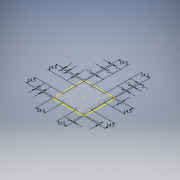
# Autodesk Inventor part: Cover
Saved by Autodesk Inventor 2016 (Build 200138000, 138)
## iProperties
Created: 2016-04-15
Part Number: Cover
Material: Generic
Document SubType Name: Modeling
Designer: Andres
Density: 1 g/cm^3
Appearance: Clear - Light
Author: Andres
Autodesk Inventor part; units mm, degrees
ref_plane "YZ Plane" through (0, 0, 0) normal (1, 0, 0) x (0, 1, 0)
ref_plane "XZ Plane" through (0, 0, 0) normal (0, 1, 0) x (-1, 0, 0)
ref_plane "XY Plane" through (0, 0, 0) normal (0, 0, 1) x (1, 0, 0)
sketch "Sketch1" plane through (0, 0, 0) normal (0, 0, 1) x (1, 0, 0)
  line L0 (-25, 25) -> (25, 25)
  line L1 (25, 25) -> (25, -25)
  line L2 (25, -25) -> (-25, -25)
  line L3 (-25, -25) -> (-25, 25)
  point P0 (0, 0)
  point P1 (-25, 0)
  point P2 (0, 25)
  dimension "d0" = 50
  dimension "d1" = 50
  constraints: 8 end point, 2 midpoint, 2 parallel, 1 horizontal, 1 horizontal alignment, 1 perpendicular, 1 vertical alignment
  measures "d0" distance of L0.end L1.end
  measures "d1" distance of L0.start L0.end
extrude "Extrusion1" add sketch "Sketch1" along normal blind 4
chamfer "Chamfer1" distance 4 distance2 2 1 edges at (0, -25, 4) measured on face at (0, -24.5, 4)
chamfer "Chamfer2" distance 4 distance2 2 1 edges at (25, 2, 4) measured on face at (24.5, 2, 4)
chamfer "Chamfer3" distance 4 distance2 2 1 edges at (-25, 2, 4) measured on face at (-24.5, 2, 4)
chamfer "Chamfer4" distance 4 distance2 2 1 edges at (0, 25, 4) measured on face at (0, 24.5, 4)
sketch "Sketch2" plane through (0, 0, 0) normal (0, 0, -1) x (-1, 0, 0)
  point P0 (0, 0)
sketch "Sketch3" plane through (0, 0, 0) normal (0, 0, -1) x (-1, 0, 0)
  point P0 (0, 0)
sketch "Sketch4" plane through (0, 0, 0) normal (0, 0, -1) x (-1, 0, 0)
  point P0 (0, 0)
sketch "Sketch5" plane through (0, 0, 0) normal (0, 0, -1) x (-1, 0, 0)
  line L0 (25, -25) -> (25, 25) projected
  line L1 (25, 25) -> (-25, 25) projected
  line L2 (-25, 25) -> (-25, -25) projected
  line L3 (-25, -25) -> (25, -25) projected
  line L4 (25, -25) -> (21, -21) projected
  point P0 (0, 0)
  point P1 (23, 23)
  point P2 (-23, 23)
  point P3 (-23, -23)
  point P4 (-23, -10.5)
  point P5 (-23, 10.5)
  point P6 (10.5, 23)
  point P7 (-10.5, 23)
  point P8 (23, 10.5)
  point P9 (23, -10.5)
  point P10 (10.5, -23)
  point P11 (-10.5, -23)
  point P12 (23, -23)
  dimension "d18" = 2
  dimension "d19" = 2
  dimension "d20" = 2
  dimension "d21" = 2
  dimension "d22" = 2
  dimension "d23" = 2
  dimension "d24" = 2
  dimension "d25" = 2
  dimension "d26" = 2
  dimension "d27" = 2
  dimension "d28" = 2
  dimension "d29" = 2
  dimension "d30" = 2
  dimension "d31" = 2
  dimension "d32" = 14.5
  dimension "d33" = 14.5
  dimension "d34" = 14.5
  dimension "d35" = 14.5
  dimension "d36" = 14.5
  dimension "d37" = 14.5
  dimension "d38" = 14.5
  dimension "d39" = 14.5
  constraints: 1 midpoint
  measures "d18" distance from line of L0 point (23, 23)
  measures "d19" distance from line of L1 point (23, 23)
  measures "d20" distance from line of L2 point (-23, 23)
  measures "d21" distance from line of L1 point (10.5, 23)
  measures "d22" distance from line of L1 point (-10.5, 23)
  measures "d23" distance from line of L1 point (-23, 23)
  measures "d24" distance from line of L0 point (23, 10.5)
  measures "d25" distance from line of L0 point (23, -10.5)
  measures "d26" distance from line of L3 point (10.5, -23)
  measures "d27" distance from line of L3 point (-10.5, -23)
  measures "d28" distance from line of L2 point (-23, 10.5)
  measures "d29" distance from line of L2 point (-23, -10.5)
  measures "d30" distance from line of L3 point (-23, -23)
  measures "d31" distance from line of L2 point (-23, -23)
  measures "d32" distance from line of L1 point (-23, 10.5)
  measures "d33" distance from line of L3 point (-23, -10.5)
  measures "d34" distance from line of L2 point (-10.5, 23)
  measures "d35" distance from line of L0 point (10.5, 23)
  measures "d36" distance from line of point (23, 10.5) L1
  measures "d37" distance from line of L3 point (23, -10.5)
  measures "d38" distance from line of L0 point (10.5, -23)
  measures "d39" distance from line of L2 point (-10.5, -23)
sketch "Sketch6" plane through (0, 0, 0) normal (0, 0, -1) x (-1, 0, 0)
  point P0 (23, 23)
  point P1 (-23, 23)
  point P2 (-23, -23)
  point P3 (-23, -10.5)
  point P4 (-23, 10.5)
  point P5 (10.5, 23)
  point P6 (-10.5, 23)
  point P7 (23, 10.5)
  point P8 (10.5, -23)
  point P9 (-10.5, -23)
  point P10 (23, -23)
  point P11 (23, -10.5)
hole "Hole1" at (-23, 23, 0) at (23, 23, 0) at (23, -23, 0) at (23, -10.5, 0) at (23, 10.5, 0) at (-10.5, 23, 0) at (10.5, 23, 0) at (-23, 10.5, 0) at (-10.5, -23, 0) at (10.5, -23, 0) at (-23, -23, 0) at (-23, -10.5, 0) direction (0, 0, 1) diameter 1.8 end up to surface
body "Solid1"
